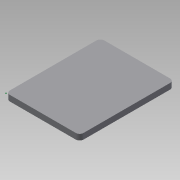
# Autodesk Inventor part: Cart_LOW_SHELF
Saved by Autodesk Inventor 2015 (Build 190159000, 159)
## iProperties
Created: 2015-05-21
Part Number: Cart_LOW_SHELF
Material: Generic
Document SubType Name: Modeling
Designer: Joe Sheldon
Density: 1 g/cm^3
Appearance: Default
Author: Joe Sheldon
Autodesk Inventor part; units mm, degrees
ref_plane "YZ Plane" through (0, 0, 0) normal (1, 0, 0) x (0, 1, 0)
ref_plane "XZ Plane" through (0, 0, 0) normal (0, 1, 0) x (-1, 0, 0)
ref_plane "XY Plane" through (0, 0, 0) normal (0, 0, 1) x (1, 0, 0)
sketch "Sketch1" plane through (0, 0, 0) normal (0, 1, 0) x (-1, 0, 0)
  line L0 (0, 0) -> (-361.95, 0)
  line L1 (-361.95, 0) -> (-361.95, -463.55)
  line L2 (-361.95, -463.55) -> (0, -463.55)
  line L3 (0, -463.55) -> (0, 0)
  dimension "d0" = 361.95
  dimension "d1" = 463.55
  constraints: 8 end point, 2 parallel, 1 horizontal, 1 perpendicular
  measures "d0" distance of L2.end L1.end
  measures "d1" distance of L1.end L0.end
extrude "Extrusion1" add sketch "Sketch1" along normal blind 2.794
fillet "Fillet1" radius 19.05 4 edges at (361.95, 1.397, 0) (361.95, 1.397, -463.55) (0, 1.397, -463.55) (0, 1.397, 0)
sketch "Sketch4" plane through (0, 0, 0) normal (0, -1, 0) x (1, 0, 0)
  point P0 (0, 0)
sketch "Sketch5" plane through (0, 0, 0) normal (0, -1, 0) x (1, 0, 0)
  arc A0 (19.05, 0) -> (0, -19.05) centre (19.05, -19.05) ccw projected
  line L0 (19.05, 0) -> (342.9, 0) projected
  line L1 (0, -444.5) -> (0, -19.05) projected
  line L2 (361.95, -19.05) -> (361.95, -444.5) projected
  arc A1 (361.95, -19.05) -> (342.9, 0) centre (342.9, -19.05) ccw projected
  arc A2 (0, -444.5) -> (19.05, -463.55) centre (19.05, -444.5) ccw projected
  line L3 (342.9, -463.55) -> (19.05, -463.55) projected
  arc A3 (342.9, -463.55) -> (361.95, -444.5) centre (342.9, -444.5) ccw projected
  arc A4 (2.9117, -444.5) -> (19.05, -460.6383) centre (19.05, -444.5) ccw
  line L4 (2.9117, -444.5) -> (2.9117, -19.05)
  arc A5 (19.05, -2.9117) -> (2.9117, -19.05) centre (19.05, -19.05) ccw
  line L5 (19.05, -2.9117) -> (342.9, -2.9117)
  arc A6 (359.0383, -19.05) -> (342.9, -2.9117) centre (342.9, -19.05) ccw
  line L6 (359.0383, -19.05) -> (359.0383, -444.5)
  arc A7 (342.9, -460.6383) -> (359.0383, -444.5) centre (342.9, -444.5) ccw
  line L7 (342.9, -460.6383) -> (19.05, -460.6383)
  point P0 (0, 0)
  constraints: 8 end point, 8 point on circle, 4 centre point, 7 other
extrude "Extrusion2" add sketch "Sketch5" along normal blind 25.4
body "Solid1"
